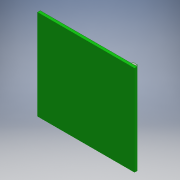
# Autodesk Inventor part: PCB Wifi
Saved by Autodesk Inventor 2019 (Build 230136000, 136)
## iProperties
Created: 2018-06-11
Part Number: PCB Wifi
Material: Nylon, disulfure de molybdène
Document SubType Name: Modeling
Designer: dimercur
Density: 1.13 g/cm^3
Appearance: Vert foncé
Mass: 8.39635 g
Surface Area: 97.36 cm^2
Volume: 7.4304 cm^3
Author: dimercur
Autodesk Inventor part; units mm, degrees
ref_plane "YZ Plane" through (0, 0, 0) normal (1, 0, 0) x (0, 1, 0)
ref_plane "XZ Plane" through (0, 0, 0) normal (0, 1, 0) x (-1, 0, 0)
ref_plane "XY Plane" through (0, 0, 0) normal (0, 0, 1) x (1, 0, 0)
sketch "Esquisse1" plane through (0, 0, 0) normal (0, 1, 0) x (-1, 0, 0)
  line L0 (28, -26) -> (-28, -26)
  line L1 (-28, -26) -> (-28, 26)
  line L2 (-28, 26) -> (28, 26)
  line L3 (28, 26) -> (28, -26)
  point P0 (0, 0)
  dimension "d0" = 56
  dimension "d1" = 28
  dimension "d2" = 52
  dimension "d3" = 26
  constraints: 8 end point, 2 parallel, 1 horizontal, 1 perpendicular
  measures "d0" distance of L0.start L0.end
  measures "d1" horizontal distance of point (0, 0) L0.start
  measures "d2" distance of L2.end L0.start
  measures "d3" vertical distance of point (0, 0) L0.start
extrude "Extrusion1" add sketch "Esquisse1" along normal blind 1.6
sketch "Esquisse2" plane through (0, 1.6, 0) normal (0, 1, 0) x (1, 0, 0)
  line L0 (-26, 24) -> (-23.5, 24)
  line L1 (-23.5, 24) -> (-23.5, -15)
  line L2 (-23.5, -15) -> (-26, -15)
  line L3 (-26, -15) -> (-26, 24)
  line L4 (22.5, 24) -> (25, 24)
  line L5 (25, 24) -> (25, -24)
  line L6 (25, -24) -> (22.5, -24)
  line L7 (22.5, -24) -> (22.5, 24)
  line L8 (28, 26) -> (-28, 26) projected
  line L9 (-28, 26) -> (-28, -26) projected
  point P0 (0, 0)
  dimension "d6" = 2.5
  dimension "d7" = 2.5
  dimension "d8" = 39
  dimension "d9" = 48
  dimension "d10" = 2
  dimension "d11" = 2
  dimension "d12" = 46
  constraints: 16 end point, 4 parallel, 2 horizontal, 2 perpendicular, 1 point on line
  measures "d6" distance of L0.start L0.end
  measures "d7" distance of L4.start L4.end
  measures "d8" distance of L2.end L0.start
  measures "d9" distance of L6.end L4.start
  measures "d10" distance between parallel lines of L8 L0
  measures "d11" distance between parallel lines of L9 L3
  measures "d12" distance between parallel lines of L7 L1
extrude "Extrusion2" add sketch "Esquisse2" along normal blind 3
equation "\"d1\" = 0.5 * d0"
equation "\"d3\" = 0.5 * d2"
